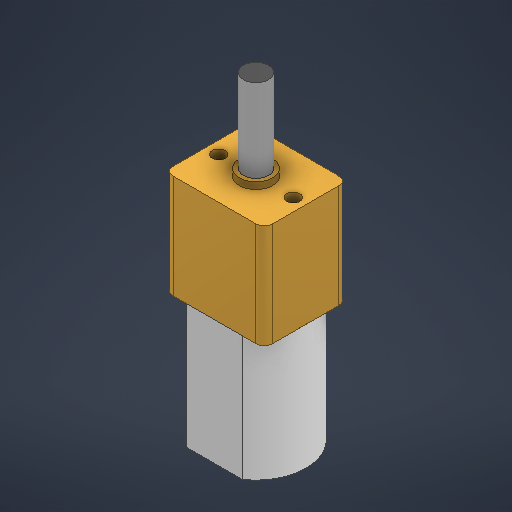
# Autodesk Inventor part: P_Gewindemotor_N20
Saved by Autodesk Inventor 2026 (Build 300175000, 175)
## iProperties
Created: 2025-04-26
Part Number: P_Gewindemotor_N20
Material: Generisch
Document SubType Name: Modeling
Designer: FAL
Density: 1 g/cm^3
Appearance: Vorgabe
Author: FAL
Autodesk Inventor part; units mm, degrees
ref_plane "YZ Plane" through (0, 0, 0) normal (1, 0, 0) x (0, 1, 0)
ref_plane "XZ Plane" through (0, 0, 0) normal (0, 1, 0) x (-1, 0, 0)
ref_plane "XY Plane" through (0, 0, 0) normal (0, 0, 1) x (1, 0, 0)
sketch "Skizze1" plane through (0, 0, 0) normal (0, 0, 1) x (1, 0, 0)
  line L0 (-6, -5) -> (6, -5)
  line L1 (6, -5) -> (6, 5)
  line L2 (6, 5) -> (-6, 5)
  line L3 (-6, 5) -> (-6, -5)
  line L4 (-6, -5) -> (6, 5) construction
  line L5 (6, -5) -> (-6, 5) construction
  point P0 (0, 0)
  dimension "d0" = 12
  dimension "d1" = 10
  constraints: 12 end point, 2 midpoint, 2 parallel, 1 horizontal, 1 perpendicular
  measures "d0" distance of L1.end L2.end
  measures "d1" distance of L0.end L1.end
extrude "Extrusion1" add sketch "Skizze1" against normal blind 12.5
sketch "Skizze2" plane through (0, 0, -12.5) normal (0, 0, -1) x (-1, 0, 0)
  line L0 (6, -5) -> (6, 5) projected
  line L1 (-3.3166, -5) -> (3.3166, -5)
  line L2 (3.3166, 5) -> (-3.3166, 5)
  line L3 (-6, -5) -> (6, 5) construction
  line L4 (6, -5) -> (-6, 5) construction
  arc A0 (3.3166, -5) -> (3.3166, 5) centre (0, 0) ccw
  arc A1 (-3.3166, 5) -> (-3.3166, -5) centre (0, 0) ccw
  line L5 (-6, 5) -> (-6, -5) projected
  line L6 (-6, -5) -> (6, -5) projected
  line L7 (6, 5) -> (-6, 5) projected
  constraints: 8 end point, 4 point on circle, 2 centre point, 2 collinear, 2 midpoint, 2 tangent, 1 coincident, 1 horizontal, 1 parallel
extrude "Extrusion2" add sketch "Skizze2" along normal blind 15 separate body contours A0 L1 A1 L2
fillet "Rundung1" radius 1 4 edges at (6, 5, -6.25) (-6, 5, -6.25) (-6, -5, -6.25) (6, -5, -6.25)
sketch "Skizze3" plane through (0, 0, 0) normal (0, 0, 1) x (1, 0, 0)
  circle A0 centre (0, 0) radius 2
  dimension "d7" = 4
  constraints: 1 centre point, 1 coincident
  measures "d7" diameter of A0
extrude "Extrusion3" add sketch "Skizze3" along normal blind 0.8 bodies 1
sketch "Skizze4" plane through (0, 0, 0.8) normal (0, 0, 1) x (1, 0, 0)
  circle A0 centre (0, 0) radius 2 projected
  circle A1 centre (0, 0) radius 1.5
  dimension "d10" = 3
  constraints: 1 centre point, 1 coincident
  measures "d10" diameter of A1
extrude "Extrusion4" add sketch "Skizze4" along normal blind 10 separate body contours A1
sketch "Skizze5" plane through (0, 0, 0) normal (0, 0, 1) x (1, 0, 0)
  line L0 (6, -4) -> (6, 4) projected
  circle A0 centre (-4.5, 0) radius 0.8
  line L1 (-4.5, 0) -> (0, 0) construction
  dimension "d15" = 1.6
  dimension "d16" = 4.5
  constraints: 2 end point, 1 centre point, 1 horizontal
  measures "d15" diameter of A0
  measures "d16" distance of L1.end L1.start
extrude "Extrusion5" cut sketch "Skizze5" against normal blind 5 bodies 1
mirror "Spiegeln1" about plane through (0, 0, 0) normal (1, 0, 0) of "Extrusion5" bodies 1
ref_plane "Arbeitsebene1" through (0, 0, 0) normal (1, 0, 0) x (0, 1, 0)
